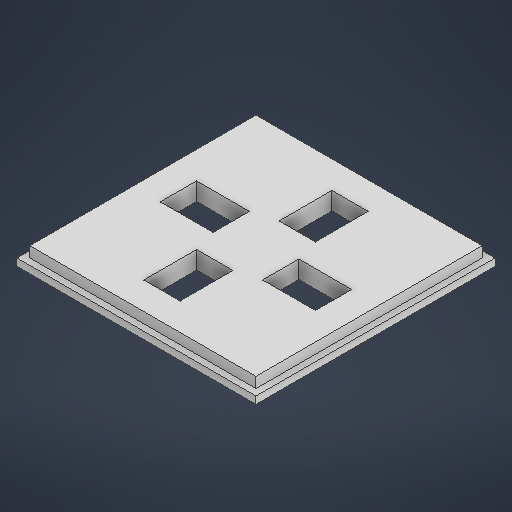
# Autodesk Inventor part: PCB_cover_platte_originaldicke
Saved by Autodesk Inventor 2026.2 (Build 302298010, 298A)
## iProperties
Created: 2026-03-12
Part Number: PCB_cover_platte_originaldicke
Material: Generisch
Document SubType Name: Modeling
Designer: ami-student
Density: 1 g/cm^3
Appearance: Vorgabe
Author: ami-student
Autodesk Inventor part; units mm, degrees
ref_plane "YZ Plane" through (0, 0, 0) normal (1, 0, 0) x (0, 1, 0)
ref_plane "XZ Plane" through (0, 0, 0) normal (0, 1, 0) x (-1, 0, 0)
ref_plane "XY Plane" through (0, 0, 0) normal (0, 0, 1) x (1, 0, 0)
sketch "Skizze1" plane through (0, 0, 0) normal (0, 0, 1) x (1, 0, 0)
  line L0 (-28.13, 28.13) -> (28.13, 28.13)
  line L1 (28.13, 28.13) -> (28.13, -28.13)
  line L2 (28.13, -28.13) -> (-28.13, -28.13)
  line L3 (-28.13, -28.13) -> (-28.13, 28.13)
  line L4 (-39.382, 0) -> (39.382, 0) construction
  line L5 (0, -39.382) -> (0, 39.382) construction
  point P0 (0, 0)
  dimension "d0" = 56.26
  constraints: 8 end point, 2 parallel, 2 perpendicular, 1 horizontal, 2 other
  measures "d0" distance of L0.start L0.end
extrude "Extrusion1" add sketch "Skizze1" along normal blind 1.7
sketch "Skizze2" plane through (0, 0, 1.7) normal (0, 0, 1) x (1, 0, 0)
  line L0 (0, -39.382) -> (0, 39.382) construction
  line L1 (-39.382, 0) -> (39.382, 0) construction
  line L2 (-26.6175, 26.6175) -> (26.6175, 26.6175)
  line L3 (26.6175, 26.6175) -> (26.6175, -26.6175)
  line L4 (26.6175, -26.6175) -> (-26.6175, -26.6175)
  line L5 (-26.6175, -26.6175) -> (-26.6175, 26.6175)
  line L6 (28.13, 28.13) -> (-28.13, 28.13) projected
  point P0 (0, 0)
  dimension "d3" = 53.235
  constraints: 8 end point, 2 parallel, 2 perpendicular, 1 horizontal, 2 other
  measures "d3" distance of L4.end L2.start
extrude "Extrusion2" add sketch "Skizze2" along normal blind 2.5
sketch "Skizze3" plane through (0, 0, 0) normal (0, 0, -1) x (-1, 0, 0)
  line L0 (28.13, -28.13) -> (-28.13, -28.13) projected
  line L1 (28.13, 28.13) -> (28.13, -28.13) projected
  line L2 (-28.13, 28.13) -> (28.13, 28.13) projected
  line L3 (-28.13, -28.13) -> (-28.13, 28.13) projected
  line L4 (-6.21, 20.195) -> (2.33, 20.195)
  line L5 (2.33, 20.195) -> (2.33, 7.76)
  line L6 (2.33, 7.76) -> (-6.21, 7.76)
  line L7 (-6.21, 7.76) -> (-6.21, 20.195)
  point P0 (0, 0)
  point P1 (0, 0)
  dimension "d6" = 21.92
  dimension "d7" = 8.54
  dimension "d8" = 12.435
  dimension "d9" = 35.89
  constraints: 8 end point, 2 parallel, 1 coincident, 1 horizontal, 1 perpendicular
  measures "d6" distance between parallel lines of L7 L3
  measures "d7" distance between parallel lines of L5 L7
  measures "d8" distance of L6.end L4.start
  measures "d9" distance between parallel lines of L6 L0
extrude "Extrusion3" cut sketch "Skizze3" against normal up to surface (4.2 mm away) contours L4 L5 L6 L7
pattern_circular "Runde Anordnung1" count 4 over 360 about axis through (0, 0, -10) along (0, 0, 1) of "Extrusion3"
sketch "Skizze4" plane through (0, 0, 0) normal (0, 0, -1) x (-1, 0, 0)
  line L0 (-28.13, -28.13) -> (-28.13, 28.13) projected
  line L1 (-28.13, 28.13) -> (28.13, 28.13) projected
  point P0 (0, 0)
  point P1 (-11.817, 11.817)
  dimension "d15" = 16.313
  dimension "d16" = 16.313
  measures "d15" distance from line of L0 point (-11.817, 11.817)
  measures "d16" distance from line of L1 point (-11.817, 11.817)
hole "Bohrung1" at (11.817, 11.817, 0) direction (0, 0, 1) diameter 5.333 depth 3.35 counterbore diameter 8.2 counterbore depth 2.2
pattern_circular "Runde Anordnung2" count 4 over 360 about axis through (0, 0, -10) along (0, 0, 1) of "Bohrung1"
sketch "Skizze5" plane through (0, 0, 0) normal (0, 0, -1) x (-1, 0, 0)
  point P0 (0, 0)
  point P1 (0, 0)
  constraints: 1 coincident
hole "Bohrung2" at (0, 0, 0) direction (0, 0, 1) diameter 5.333 depth 3.35 counterbore diameter 11.199 counterbore depth 2.2
